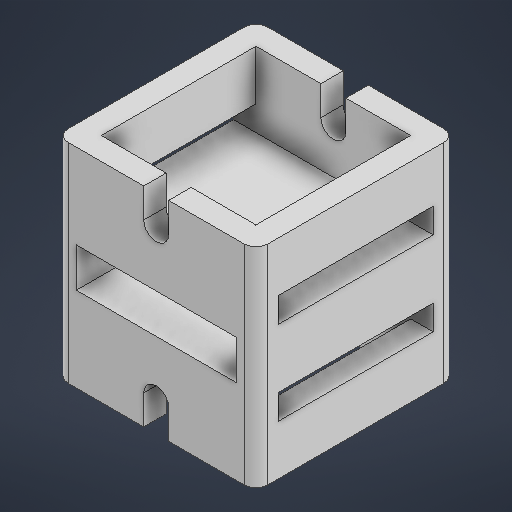
# Autodesk Inventor part: Part1
Saved by Autodesk Inventor 2026.1 (Build 301233000, 233)
## iProperties
Created: 2025-08-28
Part Number: Part1
Material: Generic
Document SubType Name: Modeling
Designer: usman
Density: 1 g/cm^3
Appearance: Default
Author: usman
Autodesk Inventor part; units mm, degrees
(part 1 of 2)
ref_plane "YZ Plane" through (0, 0, 0) normal (1, 0, 0) x (0, 1, 0)
ref_plane "XZ Plane" through (0, 0, 0) normal (0, 1, 0) x (-1, 0, 0)
ref_plane "XY Plane" through (0, 0, 0) normal (0, 0, 1) x (1, 0, 0)
sketch "Sketch1" plane through (0, 0, 0) normal (1, 0, 0) x (0, 1, 0)
  line L0 (-26.543, 25.4) -> (26.543, 25.4)
  line L1 (26.543, 25.4) -> (26.543, -25.4)
  line L2 (26.543, -25.4) -> (-26.543, -25.4)
  line L3 (-26.543, -25.4) -> (-26.543, 25.4)
  line L4 (-26.543, 25.4) -> (26.543, -25.4) construction
  line L5 (26.543, 25.4) -> (-26.543, -25.4) construction
  point P0 (0, 0)
  dimension "d0" = 53.086
  dimension "d1" = 50.8
  constraints: 12 end point, 2 midpoint, 2 parallel, 1 horizontal, 1 perpendicular
  measures "d0" distance of L1.end L2.end
  measures "d1" distance of L0.end L1.end
extrude "Extrusion1" add sketch "Sketch1" along normal blind 50.8
sketch "Sketch3" plane through (0, -26.543, -25.4) normal (0, -1, 0) x (1, 0, 0)
  line L0 (45.085, 5.715) -> (5.715, 5.715)
  line L1 (5.715, 5.715) -> (5.715, 45.085)
  line L2 (5.715, 45.085) -> (45.085, 45.085)
  line L3 (45.085, 45.085) -> (45.085, 5.715)
  line L4 (0, 0) -> (50.8, 0) projected
  line L5 (50.8, 50.8) -> (50.8, 0) projected
  point P0 (0, 25.4)
  dimension "d7" = 39.37
  dimension "d8" = 39.37
  dimension "d9" = 5.715
  dimension "d10" = 5.715
  constraints: 8 end point, 2 parallel, 1 horizontal, 1 perpendicular
  measures "d7" distance of L2.end L0.start
  measures "d8" distance of L0.start L0.end
  measures "d9" distance between parallel lines of L0 L4
  measures "d10" distance between parallel lines of L5 L3
extrude "Extrusion2" cut sketch "Sketch3" against normal blind 19.037
mirror "Mirror1" about plane through (0, 0, 0) normal (0, 1, 0) of "Extrusion2"
sketch "Sketch5" plane through (0, -26.543, 25.4) normal (0, 0, 1) x (1, 0, 0)
  line L0 (5.08, 31.543) -> (45.72, 31.543)
  line L1 (45.72, 31.543) -> (45.72, 21.543)
  line L2 (45.72, 21.543) -> (5.08, 21.543)
  line L3 (5.08, 21.543) -> (5.08, 31.543)
  line L4 (50.8, 53.086) -> (50.8, 0) projected
  line L5 (0, 53.086) -> (50.8, 53.086) projected
  point P0 (0, 26.543)
  dimension "d14" = 40.64
  dimension "d15" = 10
  dimension "d16" = 5.08
  dimension "d17" = 21.543
  constraints: 8 end point, 2 parallel, 1 horizontal, 1 perpendicular
  measures "d14" distance of L0.start L0.end
  measures "d15" distance of L2.end L0.start
  measures "d16" distance between parallel lines of L4 L1
  measures "d17" distance between parallel lines of L5 L0
extrude "Extrusion3" cut sketch "Sketch5" against normal through all
sketch "Sketch6" plane through (50.8, 0, 0) normal (1, 0, 0) x (0, 0, -1)
  line L0 (-19.685, 13.856) -> (19.685, 13.856)
  line L1 (19.685, 13.856) -> (19.685, 7.506)
  line L2 (19.685, 7.506) -> (-19.685, 7.506)
  line L3 (-19.685, 7.506) -> (-19.685, 13.856)
  line L4 (25.4, 26.543) -> (-25.4, 26.543) projected
  line L5 (-25.4, 26.543) -> (-25.4, -26.543) projected
  point P0 (0, 0)
  dimension "d20" = 39.37
  dimension "d21" = 6.35
  dimension "d22" = 12.687
  dimension "d23" = 5.715
  constraints: 8 end point, 2 parallel, 1 horizontal, 1 perpendicular
  measures "d20" distance of L0.start L0.end
  measures "d21" distance of L0.end L1.end
  measures "d22" distance between parallel lines of L4 L0
  measures "d23" distance between parallel lines of L5 L3
extrude "Extrusion4" cut sketch "Sketch6" against normal through all
mirror "Mirror2" about plane through (0, 0, 0) normal (0, 1, 0) of "Extrusion4"
sketch "Sketch7" plane through (0, -26.543, -25.4) normal (0, 0, -1) x (-1, 0, 0)
  line L0 (0, 53.086) -> (-50.8, 53.086) projected
  line L1 (-22.225, 53.086) -> (-22.225, 45.593)
  line L2 (-28.575, 53.086) -> (-28.575, 45.593)
  arc A0 (-28.575, 45.593) -> (-22.225, 45.593) centre (-25.4, 45.593) ccw
  point P0 (0, 26.543)
  point P1 (-25.4, 53.086)
  dimension "d26" = 7.493
  dimension "d27" = 7.493
  dimension "d28" = 3.175
  dimension "d29" = 3.175
  constraints: 4 end point, 2 point on circle, 2 point on line, 1 centre point, 1 midpoint, 1 perpendicular, 1 tangent, 1 vertical
  measures "d26" distance of L2.start L2.end
  measures "d27" distance of L1.start L1.end
  measures "d28" distance from line of L1 point (-25.4, 53.086)
  measures "d29" distance from line of point (-25.4, 53.086) L2
extrude "Extrusion5" cut sketch "Sketch7" against normal through all
mirror "Mirror3" about plane through (0, 0, 0) normal (0, 1, 0) of "Extrusion5"
fillet "Fillet2" radius 3 4 edges at (0, 0, -25.4) (0, 0, 25.4) (50.8, 0, -25.4) (50.8, 0, 25.4)
sketch "Sketch8" plane through (25.4, 19.05, -25.4) normal (0, 0, -1) x (-1, 0, 0)
  line L0 (-22.3221, -6.5134) -> (22.2832, -6.5134) construction
  line L1 (22.2832, -6.5134) -> (22.2832, -12.0545) construction
  line L2 (22.2832, -12.0545) -> (-22.3221, -12.0545) construction
  line L3 (-22.3221, -12.0545) -> (-22.3221, -6.5134) construction
  line L4 (-22.2875, -25.5953) -> (22.4563, -25.5953) construction
  line L5 (22.4563, -25.5953) -> (22.4563, -34.5995) construction
  line L6 (22.4563, -34.5995) -> (-22.2875, -34.5995) construction
  line L7 (-22.2875, -34.5995) -> (-22.2875, -25.5953) construction
  spline S0 degree 2 poles (-17.6545, -8.2254) (-17.325, -8.2955) (-17.1616, -8.4511) knots 0 0 0 1 1 1
  spline S1 degree 2 poles (-17.1616, -8.4511) (-16.9333, -8.6638) (-16.9333, -8.9751) knots 0 0 0 1 1 1
  spline S2 degree 2 poles (-16.9333, -8.9751) (-16.9333, -9.2111) (-17.2342, -9.6443) (-17.7556, -9.8441) (-18.2926, -9.8441) knots 0 0 0 1 2 3 3 3
  line L8 (-18.2926, -9.8441) -> (-19.7919, -9.8441)
  line L9 (-19.7919, -9.8441) -> (-19.7919, -9.7585)
  line L10 (-19.7919, -9.7585) -> (-19.6726, -9.7585)
  spline S3 degree 2 poles (-19.6726, -9.7585) (-19.4728, -9.7585) (-19.3872, -9.6314) knots 0 0 0 1 1 1
  spline S4 degree 2 poles (-19.3872, -9.6314) (-19.3328, -9.5483) (-19.3328, -9.2812) knots 0 0 0 1 1 1
  line L11 (-19.3328, -9.2812) -> (-19.3328, -7.2319)
  spline S5 degree 2 poles (-19.3328, -7.2319) (-19.3328, -6.9362) (-19.4002, -6.8584) knots 0 0 0 1 1 1
  spline S6 degree 2 poles (-19.4002, -6.8584) (-19.491, -6.7547) (-19.6726, -6.7547) knots 0 0 0 1 1 1
  line L12 (-19.6726, -6.7547) -> (-19.7919, -6.7547)
  line L13 (-19.7919, -6.7547) -> (-19.7919, -6.6691)
  line L14 (-19.7919, -6.6691) -> (-18.4197, -6.6691)
  spline S7 degree 2 poles (-18.4197, -6.6691) (-18.0358, -6.6691) (-17.8023, -6.7261) knots 0 0 0 1 1 1
  spline S8 degree 2 poles (-17.8023, -6.7261) (-17.4521, -6.8091) (-17.0812, -7.2397) (-17.0812, -7.5173) knots 0 0 0 1 2 2 2
  spline S9 degree 2 poles (-17.0812, -7.5173) (-17.0812, -7.7559) (-17.3717, -8.1346) (-17.6545, -8.2254) knots 0 0 0 1 2 2 2
  spline S10 degree 2 poles (-18.884, -9.6158) (-18.6116, -9.678) (-18.3445, -9.678) knots 0 0 0 1 1 1
  spline S11 degree 2 poles (-18.3445, -9.678) (-17.9191, -9.678) (-17.4703, -9.2967) (-17.4703, -9.0166) knots 0 0 0 1 2 2 2
  spline S12 degree 2 poles (-17.4703, -9.0166) (-17.4703, -8.8298) (-17.6778, -8.49) (-18.1344, -8.2929) (-18.469, -8.2929) knots 0 0 0 1 2 3 3 3
  spline S13 degree 2 poles (-18.469, -8.2929) (-18.6142, -8.2929) (-18.8217, -8.3033) (-18.884, -8.3136) knots 0 0 0 1 2 2 2
  line L15 (-18.884, -8.3136) -> (-18.884, -9.6158)
  spline S14 degree 2 poles (-18.884, -8.0983) (-18.7984, -8.1165) (-18.5753, -8.132) (-18.4404, -8.132) knots 0 0 0 1 2 2 2
  spline S15 degree 2 poles (-18.4404, -8.132) (-18.098, -8.132) (-17.753, -7.9842) (-17.5715, -7.6781) (-17.5715, -7.4991) knots 0 0 0 1 2 3 3 3
  spline S16 degree 2 poles (-17.5715, -7.4991) (-17.5715, -7.219) (-18.0254, -6.8247) (-18.4612, -6.8247) knots 0 0 0 1 2 2 2
  spline S17 degree 2 poles (-18.4612, -6.8247) (-18.6972, -6.8247) (-18.884, -6.8766) knots 0 0 0 1 1 1
  line L16 (-18.884, -6.8766) -> (-18.884, -8.0983)
  spline S18 degree 2 poles (-15.3095, -9.5328) (-15.639, -9.7896) (-15.7246, -9.8285) knots 0 0 0 1 1 1
  spline S19 degree 2 poles (-15.7246, -9.8285) (-15.8491, -9.8882) (-15.9917, -9.8882) knots 0 0 0 1 1 1
  spline S20 degree 2 poles (-15.9917, -9.8882) (-16.2148, -9.8882) (-16.5028, -9.5847) (-16.5028, -9.3356) knots 0 0 0 1 2 2 2
  spline S21 degree 2 poles (-16.5028, -9.3356) (-16.5028, -9.18) (-16.4327, -9.0633) knots 0 0 0 1 1 1
  spline S22 degree 2 poles (-16.4327, -9.0633) (-16.3367, -8.905) (-15.862, -8.6249) (-15.3095, -8.4226) knots 0 0 0 1 2 2 2
  line L17 (-15.3095, -8.4226) -> (-15.3095, -8.3396)
  spline S23 degree 2 poles (-15.3095, -8.3396) (-15.3095, -8.0179) (-15.5119, -7.7793) (-15.7064, -7.7793) knots 0 0 0 1 2 2 2
  spline S24 degree 2 poles (-15.7064, -7.7793) (-15.8517, -7.7793) (-15.9399, -7.8597) knots 0 0 0 1 1 1
  spline S25 degree 2 poles (-15.9399, -7.8597) (-16.0281, -7.9375) (-16.0281, -8.0413) knots 0 0 0 1 1 1
  line L18 (-16.0281, -8.0413) -> (-16.0229, -8.1761)
  spline S26 degree 2 poles (-16.0229, -8.1761) (-16.0229, -8.2851) (-16.1344, -8.4018) (-16.2226, -8.4018) knots 0 0 0 1 2 2 2
  spline S27 degree 2 poles (-16.2226, -8.4018) (-16.3082, -8.4018) (-16.4197, -8.2799) (-16.4197, -8.1736) knots 0 0 0 1 2 2 2
  spline S28 degree 2 poles (-16.4197, -8.1736) (-16.4197, -7.9738) (-16.0073, -7.6366) (-15.6364, -7.6366) knots 0 0 0 1 2 2 2
  spline S29 degree 2 poles (-15.6364, -7.6366) (-15.351, -7.6366) (-15.1695, -7.7326) knots 0 0 0 1 1 1
  spline S30 degree 2 poles (-15.1695, -7.7326) (-15.0294, -7.8052) (-14.9645, -7.9583) knots 0 0 0 1 1 1
  spline S31 degree 2 poles (-14.9645, -7.9583) (-14.923, -8.0594) (-14.923, -8.3707) knots 0 0 0 1 1 1
  line L19 (-14.923, -8.3707) -> (-14.923, -9.0996)
  spline S32 degree 2 poles (-14.923, -9.0996) (-14.923, -9.4057) (-14.8997, -9.5432) (-14.8452, -9.5899) (-14.8115, -9.5899) knots 0 0 0 1 2 3 3 3
  spline S33 degree 2 poles (-14.8115, -9.5899) (-14.7726, -9.5899) (-14.7441, -9.5743) knots 0 0 0 1 1 1
  spline S34 degree 2 poles (-14.7441, -9.5743) (-14.6948, -9.5432) (-14.5547, -9.4031) knots 0 0 0 1 1 1
  line L20 (-14.5547, -9.4031) -> (-14.5547, -9.5328)
  spline S35 degree 2 poles (-14.5547, -9.5328) (-14.8167, -9.8856) (-15.0553, -9.8856) knots 0 0 0 1 1 1
  spline S36 degree 2 poles (-15.0553, -9.8856) (-15.1721, -9.8856) (-15.3069, -9.7273) (-15.3095, -9.5328) knots 0 0 0 1 2 2 2
  line L21 (-15.3095, -9.3823) -> (-15.3095, -8.5652)
  spline S37 degree 2 poles (-15.3095, -8.5652) (-15.6623, -8.7053) (-15.7661, -8.765) knots 0 0 0 1 1 1
  spline S38 degree 2 poles (-15.7661, -8.765) (-15.9502, -8.8661) (-16.1085, -9.0918) (-16.1085, -9.2241) knots 0 0 0 1 2 2 2
  spline S39 degree 2 poles (-16.1085, -9.2241) (-16.1085, -9.3927) (-15.9087, -9.6158) (-15.7764, -9.6158) knots 0 0 0 1 2 2 2
  spline S40 degree 2 poles (-15.7764, -9.6158) (-15.6001, -9.6158) (-15.3095, -9.3823) knots 0 0 0 1 1 1
  line L22 (-13.0087, -7.6366) -> (-13.0087, -8.3681)
  line L23 (-13.0087, -8.3681) -> (-13.0865, -8.3681)
  spline S41 degree 2 poles (-13.0865, -8.3681) (-13.1747, -8.0231) (-13.4523, -7.7741) (-13.6676, -7.7741) knots 0 0 0 1 2 2 2
  spline S42 degree 2 poles (-13.6676, -7.7741) (-13.831, -7.7741) (-14.0333, -7.9479) (-14.0333, -8.0516) knots 0 0 0 1 2 2 2
  spline S43 degree 2 poles (-14.0333, -8.0516) (-14.0333, -8.1839) (-13.9581, -8.2773) knots 0 0 0 1 1 1
  spline S44 degree 2 poles (-13.9581, -8.2773) (-13.888, -8.3733) (-13.665, -8.4822) knots 0 0 0 1 1 1
  line L24 (-13.665, -8.4822) -> (-13.3226, -8.6482)
  spline S45 degree 2 poles (-13.3226, -8.6482) (-12.8479, -8.8791) (-12.8479, -9.2578) knots 0 0 0 1 1 1
  spline S46 degree 2 poles (-12.8479, -9.2578) (-12.8479, -9.5509) (-13.2888, -9.9089) (-13.5638, -9.9089) knots 0 0 0 1 2 2 2
  spline S47 degree 2 poles (-13.5638, -9.9089) (-13.7609, -9.9089) (-14.0126, -9.8389) knots 0 0 0 1 1 1
  spline S48 degree 2 poles (-14.0126, -9.8389) (-14.0904, -9.8155) (-14.1397, -9.8155) knots 0 0 0 1 1 1
  spline S49 degree 2 poles (-14.1397, -9.8155) (-14.1915, -9.8155) (-14.2227, -9.8752) knots 0 0 0 1 1 1
  line L25 (-14.2227, -9.8752) -> (-14.3005, -9.8752)
  line L26 (-14.3005, -9.8752) -> (-14.3005, -9.11)
  line L27 (-14.3005, -9.11) -> (-14.2227, -9.11)
  spline S50 degree 2 poles (-14.2227, -9.11) (-14.1578, -9.4394) (-13.7895, -9.7714) (-13.5586, -9.7714) knots 0 0 0 1 2 2 2
  spline S51 degree 2 poles (-13.5586, -9.7714) (-13.3978, -9.7714) (-13.1955, -9.5821) (-13.1955, -9.4472) knots 0 0 0 1 2 2 2
  spline S52 degree 2 poles (-13.1955, -9.4472) (-13.1955, -9.2864) (-13.4211, -9.0659) (-14.1008, -8.7313) (-14.2071, -8.5938) knots 0 0 0 1 2 3 3 3
  spline S53 degree 2 poles (-14.2071, -8.5938) (-14.3109, -8.4615) (-14.3109, -8.2566) knots 0 0 0 1 1 1
  spline S54 degree 2 poles (-14.3109, -8.2566) (-14.3109, -7.992) (-13.9477, -7.6366) (-13.6598, -7.6366) knots 0 0 0 1 2 2 2
  spline S55 degree 2 poles (-13.6598, -7.6366) (-13.5327, -7.6366) (-13.3537, -7.6911) knots 0 0 0 1 1 1
  spline S56 degree 2 poles (-13.3537, -7.6911) (-13.2344, -7.7248) (-13.1955, -7.7248) knots 0 0 0 1 1 1
  spline S57 degree 2 poles (-13.1955, -7.7248) (-13.1566, -7.7248) (-13.115, -7.6911) (-13.0865, -7.6366) knots 0 0 0 1 2 2 2
  line L28 (-13.0865, -7.6366) -> (-13.0087, -7.6366)
  spline S58 degree 2 poles (-12.1657, -8.5082) (-12.1683, -8.9855) (-11.9348, -9.2552) knots 0 0 0 1 1 1
  spline S59 degree 2 poles (-11.9348, -9.2552) (-11.6988, -9.5276) (-11.3823, -9.5276) knots 0 0 0 1 1 1
  spline S60 degree 2 poles (-11.3823, -9.5276) (-11.1722, -9.5276) (-10.8609, -9.2967) (-10.7546, -9.014) knots 0 0 0 1 2 2 2
  line L29 (-10.7546, -9.014) -> (-10.6819, -9.0607)
  spline S61 degree 2 poles (-10.6819, -9.0607) (-10.7312, -9.3823) (-11.2033, -9.9089) (-11.5613, -9.9089) knots 0 0 0 1 2 2 2
  spline S62 degree 2 poles (-11.5613, -9.9089) (-11.9478, -9.9089) (-12.4977, -9.3071) (-12.4977, -8.8013) knots 0 0 0 1 2 2 2
  spline S63 degree 2 poles (-12.4977, -8.8013) (-12.4977, -8.2514) (-11.9322, -7.6366) (-11.5068, -7.6366) knots 0 0 0 1 2 2 2
  spline S64 degree 2 poles (-11.5068, -7.6366) (-11.1462, -7.6366) (-10.6819, -8.1113) (-10.6819, -8.5082) knots 0 0 0 1 2 2 2
  line L30 (-10.6819, -8.5082) -> (-12.1657, -8.5082)
  line L31 (-12.1657, -8.3733) -> (-11.1696, -8.3733)
  spline S65 degree 2 poles (-11.1696, -8.3733) (-11.1826, -8.1684) (-11.2189, -8.0828) knots 0 0 0 1 1 1
  spline S66 degree 2 poles (-11.2189, -8.0828) (-11.2785, -7.9531) (-11.5094, -7.8026) (-11.6365, -7.8026) knots 0 0 0 1 2 2 2
  spline S67 degree 2 poles (-11.6365, -7.8026) (-11.831, -7.8026) (-12.1397, -8.1035) (-12.1657, -8.3733) knots 0 0 0 1 2 2 2
  line L32 (-7.385, -9.8441) -> (-8.6145, -7.1723)
  line L33 (-8.6145, -7.1723) -> (-8.6145, -9.2941)
  spline S68 degree 2 poles (-8.6145, -9.2941) (-8.6145, -9.5873) (-8.5523, -9.6599) knots 0 0 0 1 1 1
  spline S69 degree 2 poles (-8.5523, -9.6599) (-8.4641, -9.7585) (-8.2773, -9.7585) knots 0 0 0 1 1 1
  line L34 (-8.2773, -9.7585) -> (-8.1658, -9.7585)
  line L35 (-8.1658, -9.7585) -> (-8.1658, -9.8441)
  line L36 (-8.1658, -9.8441) -> (-9.2682, -9.8441)
  line L37 (-9.2682, -9.8441) -> (-9.2682, -9.7585)
  line L38 (-9.2682, -9.7585) -> (-9.1567, -9.7585)
  spline S70 degree 2 poles (-9.1567, -9.7585) (-8.9543, -9.7585) (-8.8713, -9.6365) knots 0 0 0 1 1 1
  spline S71 degree 2 poles (-8.8713, -9.6365) (-8.8195, -9.5613) (-8.8195, -9.2941) knots 0 0 0 1 1 1
  line L39 (-8.8195, -9.2941) -> (-8.8195, -7.219)
  spline S72 degree 2 poles (-8.8195, -7.219) (-8.8195, -7.0089) (-8.8662, -6.9129) knots 0 0 0 1 1 1
  spline S73 degree 2 poles (-8.8662, -6.9129) (-8.8999, -6.8454) (-9.0737, -6.7547) (-9.2682, -6.7547) knots 0 0 0 1 2 2 2
  line L40 (-9.2682, -6.7547) -> (-9.2682, -6.6691)
  line L41 (-9.2682, -6.6691) -> (-8.3681, -6.6691)
  line L42 (-8.3681, -6.6691) -> (-7.2164, -9.1541)
  line L43 (-7.2164, -9.1541) -> (-6.0802, -6.6691)
  line L44 (-6.0802, -6.6691) -> (-5.1853, -6.6691)
  line L45 (-5.1853, -6.6691) -> (-5.1853, -6.7547)
  line L46 (-5.1853, -6.7547) -> (-5.2943, -6.7547)
  spline S74 degree 2 poles (-5.2943, -6.7547) (-5.4992, -6.7547) (-5.5822, -6.8766) knots 0 0 0 1 1 1
  spline S75 degree 2 poles (-5.5822, -6.8766) (-5.6341, -6.9518) (-5.6341, -7.219) knots 0 0 0 1 1 1
  line L47 (-5.6341, -7.219) -> (-5.6341, -9.2941)
  spline S76 degree 2 poles (-5.6341, -9.2941) (-5.6341, -9.5873) (-5.5692, -9.6599) knots 0 0 0 1 1 1
  spline S77 degree 2 poles (-5.5692, -9.6599) (-5.481, -9.7585) (-5.2943, -9.7585) knots 0 0 0 1 1 1
  line L48 (-5.2943, -9.7585) -> (-5.1853, -9.7585)
  line L49 (-5.1853, -9.7585) -> (-5.1853, -9.8441)
  line L50 (-5.1853, -9.8441) -> (-6.5316, -9.8441)
  line L51 (-6.5316, -9.8441) -> (-6.5316, -9.7585)
  line L52 (-6.5316, -9.7585) -> (-6.4201, -9.7585)
  spline S78 degree 2 poles (-6.4201, -9.7585) (-6.2151, -9.7585) (-6.1347, -9.6365) knots 0 0 0 1 1 1
  spline S79 degree 2 poles (-6.1347, -9.6365) (-6.0828, -9.5613) (-6.0828, -9.2941) knots 0 0 0 1 1 1
  line L53 (-6.0828, -9.2941) -> (-6.0828, -7.1723)
  line L54 (-6.0828, -7.1723) -> (-7.3072, -9.8441)
  line L55 (-7.3072, -9.8441) -> (-7.385, -9.8441)
  spline S80 degree 2 poles (-3.7197, -9.5328) (-4.0492, -9.7896) (-4.1348, -9.8285) knots 0 0 0 1 1 1
  spline S81 degree 2 poles (-4.1348, -9.8285) (-4.2593, -9.8882) (-4.402, -9.8882) knots 0 0 0 1 1 1
  spline S82 degree 2 poles (-4.402, -9.8882) (-4.625, -9.8882) (-4.913, -9.5847) (-4.913, -9.3356) knots 0 0 0 1 2 2 2
  spline S83 degree 2 poles (-4.913, -9.3356) (-4.913, -9.18) (-4.8429, -9.0633) knots 0 0 0 1 1 1
  spline S84 degree 2 poles (-4.8429, -9.0633) (-4.747, -8.905) (-4.2723, -8.6249) (-3.7197, -8.4226) knots 0 0 0 1 2 2 2
  line L56 (-3.7197, -8.4226) -> (-3.7197, -8.3396)
  spline S85 degree 2 poles (-3.7197, -8.3396) (-3.7197, -8.0179) (-3.9221, -7.7793) (-4.1166, -7.7793) knots 0 0 0 1 2 2 2
  spline S86 degree 2 poles (-4.1166, -7.7793) (-4.2619, -7.7793) (-4.3501, -7.8597) knots 0 0 0 1 1 1
  spline S87 degree 2 poles (-4.3501, -7.8597) (-4.4383, -7.9375) (-4.4383, -8.0413) knots 0 0 0 1 1 1
  line L57 (-4.4383, -8.0413) -> (-4.4331, -8.1761)
  spline S88 degree 2 poles (-4.4331, -8.1761) (-4.4331, -8.2851) (-4.5446, -8.4018) (-4.6328, -8.4018) knots 0 0 0 1 2 2 2
  spline S89 degree 2 poles (-4.6328, -8.4018) (-4.7184, -8.4018) (-4.83, -8.2799) (-4.83, -8.1736) knots 0 0 0 1 2 2 2
  spline S90 degree 2 poles (-4.83, -8.1736) (-4.83, -7.9738) (-4.4175, -7.6366) (-4.0466, -7.6366) knots 0 0 0 1 2 2 2
  spline S91 degree 2 poles (-4.0466, -7.6366) (-3.7613, -7.6366) (-3.5797, -7.7326) knots 0 0 0 1 1 1
  spline S92 degree 2 poles (-3.5797, -7.7326) (-3.4396, -7.8052) (-3.3748, -7.9583) knots 0 0 0 1 1 1
  spline S93 degree 2 poles (-3.3748, -7.9583) (-3.3332, -8.0594) (-3.3332, -8.3707) knots 0 0 0 1 1 1
  line L58 (-3.3332, -8.3707) -> (-3.3332, -9.0996)
  spline S94 degree 2 poles (-3.3332, -9.0996) (-3.3332, -9.4057) (-3.3099, -9.5432) (-3.2554, -9.5899) (-3.2217, -9.5899) knots 0 0 0 1 2 3 3 3
  spline S95 degree 2 poles (-3.2217, -9.5899) (-3.1828, -9.5899) (-3.1543, -9.5743) knots 0 0 0 1 1 1
  spline S96 degree 2 poles (-3.1543, -9.5743) (-3.105, -9.5432) (-2.9649, -9.4031) knots 0 0 0 1 1 1
  line L59 (-2.9649, -9.4031) -> (-2.9649, -9.5328)
  spline S97 degree 2 poles (-2.9649, -9.5328) (-3.2269, -9.8856) (-3.4655, -9.8856) knots 0 0 0 1 1 1
  spline S98 degree 2 poles (-3.4655, -9.8856) (-3.5823, -9.8856) (-3.7172, -9.7273) (-3.7197, -9.5328) knots 0 0 0 1 2 2 2
  line L60 (-3.7197, -9.3823) -> (-3.7197, -8.5652)
  spline S99 degree 2 poles (-3.7197, -8.5652) (-4.0725, -8.7053) (-4.1763, -8.765) knots 0 0 0 1 1 1
  spline S100 degree 2 poles (-4.1763, -8.765) (-4.3605, -8.8661) (-4.5187, -9.0918) (-4.5187, -9.2241) knots 0 0 0 1 2 2 2
  spline S101 degree 2 poles (-4.5187, -9.2241) (-4.5187, -9.3927) (-4.319, -9.6158) (-4.1867, -9.6158) knots 0 0 0 1 2 2 2
  spline S102 degree 2 poles (-4.1867, -9.6158) (-4.0103, -9.6158) (-3.7197, -9.3823) knots 0 0 0 1 1 1
  spline S103 degree 2 poles (-2.2308, -9.0607) (-2.428, -8.9647) (-2.6381, -8.6223) (-2.6381, -8.4122) knots 0 0 0 1 2 2 2
  spline S104 degree 2 poles (-2.6381, -8.4122) (-2.6381, -8.0957) (-2.1582, -7.6366) (-1.7821, -7.6366) knots 0 0 0 1 2 2 2
  spline S105 degree 2 poles (-1.7821, -7.6366) (-1.476, -7.6366) (-1.2503, -7.7871) knots 0 0 0 1 1 1
  line L61 (-1.2503, -7.7871) -> (-0.7964, -7.7871)
  spline S106 degree 2 poles (-0.7964, -7.7871) (-0.6952, -7.7871) (-0.6615, -7.7974) (-0.6537, -7.813) knots 0 0 0 1 2 2 2
  spline S107 degree 2 poles (-0.6537, -7.813) (-0.6407, -7.8337) (-0.6407, -7.8882) knots 0 0 0 1 1 1
  spline S108 degree 2 poles (-0.6407, -7.8882) (-0.6407, -7.9479) (-0.6537, -7.9712) knots 0 0 0 1 1 1
  spline S109 degree 2 poles (-0.6537, -7.9712) (-0.6589, -7.9842) (-0.6952, -7.9972) (-0.7964, -7.9972) knots 0 0 0 1 2 2 2
  line L62 (-0.7964, -7.9972) -> (-1.0765, -7.9972)
  spline S110 degree 2 poles (-1.0765, -7.9972) (-0.9442, -8.1658) (-0.9442, -8.4278) knots 0 0 0 1 1 1
  spline S111 degree 2 poles (-0.9442, -8.4278) (-0.9442, -8.7287) (-1.4033, -9.1541) (-1.7898, -9.1541) knots 0 0 0 1 2 2 2
  spline S112 degree 2 poles (-1.7898, -9.1541) (-1.9481, -9.1541) (-2.1167, -9.1074) knots 0 0 0 1 1 1
  spline S113 degree 2 poles (-2.1167, -9.1074) (-2.2178, -9.1956) (-2.2905, -9.3279) (-2.2905, -9.3746) knots 0 0 0 1 2 2 2
  spline S114 degree 2 poles (-2.2905, -9.3746) (-2.2905, -9.4161) (-2.2127, -9.4913) (-2.1011, -9.5068) knots 0 0 0 1 2 2 2
  spline S115 degree 2 poles (-2.1011, -9.5068) (-2.0363, -9.5172) (-1.7717, -9.5224) knots 0 0 0 1 1 1
  spline S116 degree 2 poles (-1.7717, -9.5224) (-1.2892, -9.5354) (-1.1465, -9.5561) knots 0 0 0 1 1 1
  spline S117 degree 2 poles (-1.1465, -9.5561) (-0.9287, -9.5873) (-0.6693, -9.8492) (-0.6693, -10.0386) knots 0 0 0 1 2 2 2
  spline S118 degree 2 poles (-0.6693, -10.0386) (-0.6693, -10.3032) (-0.9183, -10.5341) knots 0 0 0 1 1 1
  spline S119 degree 2 poles (-0.9183, -10.5341) (-1.284, -10.8765) (-1.8729, -10.8765) knots 0 0 0 1 1 1
  spline S120 degree 2 poles (-1.8729, -10.8765) (-2.3242, -10.8765) (-2.6355, -10.6741) knots 0 0 0 1 1 1
  spline S121 degree 2 poles (-2.6355, -10.6741) (-2.8119, -10.5574) (-2.8119, -10.4303) knots 0 0 0 1 1 1
  spline S122 degree 2 poles (-2.8119, -10.4303) (-2.8119, -10.3732) (-2.7859, -10.3188) knots 0 0 0 1 1 1
  spline S123 degree 2 poles (-2.7859, -10.3188) (-2.747, -10.2306) (-2.6225, -10.0775) knots 0 0 0 1 1 1
  spline S124 degree 2 poles (-2.6225, -10.0775) (-2.6043, -10.0568) (-2.3839, -9.8259) knots 0 0 0 1 1 1
  spline S125 degree 2 poles (-2.3839, -9.8259) (-2.5032, -9.7533) (-2.6043, -9.6365) (-2.6043, -9.5639) knots 0 0 0 1 2 2 2
  spline S126 degree 2 poles (-2.6043, -9.5639) (-2.6043, -9.4835) (-2.4721, -9.263) (-2.2308, -9.0607) knots 0 0 0 1 2 2 2
  spline S127 degree 2 poles (-2.2542, -9.8441) (-2.3657, -9.9634) (-2.4772, -10.1683) (-2.4772, -10.2539) knots 0 0 0 1 2 2 2
  spline S128 degree 2 poles (-2.4772, -10.2539) (-2.4772, -10.3654) (-2.3424, -10.4485) knots 0 0 0 1 1 1
  spline S129 degree 2 poles (-2.3424, -10.4485) (-2.1063, -10.5937) (-1.6627, -10.5937) knots 0 0 0 1 1 1
  spline S130 degree 2 poles (-1.6627, -10.5937) (-1.2425, -10.5937) (-0.8405, -10.298) (-0.8405, -10.132) knots 0 0 0 1 2 2 2
  spline S131 degree 2 poles (-0.8405, -10.132) (-0.8405, -10.0101) (-0.9598, -9.9582) knots 0 0 0 1 1 1
  spline S132 degree 2 poles (-0.9598, -9.9582) (-1.0817, -9.9089) (-1.4423, -9.8985) knots 0 0 0 1 1 1
  spline S133 degree 2 poles (-1.4423, -9.8985) (-1.9714, -9.8856) (-2.2542, -9.8441) knots 0 0 0 1 1 1
  spline S134 degree 2 poles (-1.8236, -7.7481) (-1.9974, -7.7481) (-2.2308, -8.0231) (-2.2308, -8.3084) knots 0 0 0 1 2 2 2
  spline S135 degree 2 poles (-2.2308, -8.3084) (-2.2308, -8.6794) (-2.0726, -8.8817) knots 0 0 0 1 1 1
  spline S136 degree 2 poles (-2.0726, -8.8817) (-1.9507, -9.0373) (-1.7613, -9.0373) knots 0 0 0 1 1 1
  spline S137 degree 2 poles (-1.7613, -9.0373) (-1.5849, -9.0373) (-1.3541, -8.7702) (-1.3541, -8.4848) knots 0 0 0 1 2 2 2
  spline S138 degree 2 poles (-1.3541, -8.4848) (-1.3541, -8.1139) (-1.5149, -7.9038) knots 0 0 0 1 1 1
  spline S139 degree 2 poles (-1.5149, -7.9038) (-1.6342, -7.7481) (-1.8236, -7.7481) knots 0 0 0 1 1 1
  spline S140 degree 2 poles (0.2231, -8.0905) (0.5992, -7.6366) (0.9416, -7.6366) knots 0 0 0 1 1 1
  spline S141 degree 2 poles (0.9416, -7.6366) (1.1154, -7.6366) (1.367, -7.813) (1.4422, -8.0127) knots 0 0 0 1 2 2 2
  spline S142 degree 2 poles (1.4422, -8.0127) (1.4941, -8.1528) (1.4941, -8.4433) knots 0 0 0 1 1 1
  line L63 (1.4941, -8.4433) -> (1.4941, -9.359)
  spline S143 degree 2 poles (1.4941, -9.359) (1.4941, -9.5613) (1.5278, -9.6339) knots 0 0 0 1 1 1
  spline S144 degree 2 poles (1.5278, -9.6339) (1.5538, -9.6936) (1.6679, -9.7585) (1.8209, -9.7585) knots 0 0 0 1 2 2 2
  line L64 (1.8209, -9.7585) -> (1.8209, -9.8441)
  line L65 (1.8209, -9.8441) -> (0.7574, -9.8441)
  line L66 (0.7574, -9.8441) -> (0.7574, -9.7585)
  line L67 (0.7574, -9.7585) -> (0.8015, -9.7585)
  spline S145 degree 2 poles (0.8015, -9.7585) (0.952, -9.7585) (1.0713, -9.6677) (1.0946, -9.5795) knots 0 0 0 1 2 2 2
  spline S146 degree 2 poles (1.0946, -9.5795) (1.105, -9.5432) (1.105, -9.359) knots 0 0 0 1 1 1
  line L68 (1.105, -9.359) -> (1.105, -8.4822)
  spline S147 degree 2 poles (1.105, -8.4822) (1.105, -8.1891) (0.9546, -7.9245) (0.7756, -7.9245) knots 0 0 0 1 2 2 2
  spline S148 degree 2 poles (0.7756, -7.9245) (0.498, -7.9245) (0.2231, -8.228) knots 0 0 0 1 1 1
  line L69 (0.2231, -8.228) -> (0.2231, -9.359)
  spline S149 degree 2 poles (0.2231, -9.359) (0.2231, -9.5769) (0.249, -9.6288) knots 0 0 0 1 1 1
  spline S150 degree 2 poles (0.249, -9.6288) (0.2827, -9.6962) (0.3969, -9.7585) (0.5732, -9.7585) knots 0 0 0 1 2 2 2
  line L70 (0.5732, -9.7585) -> (0.5732, -9.8441)
  line L71 (0.5732, -9.8441) -> (-0.4929, -9.8441)
  line L72 (-0.4929, -9.8441) -> (-0.4929, -9.7585)
  line L73 (-0.4929, -9.7585) -> (-0.4462, -9.7585)
  spline S151 degree 2 poles (-0.4462, -9.7585) (-0.2802, -9.7585) (-0.166, -9.5924) (-0.166, -9.359) knots 0 0 0 1 2 2 2
  line L74 (-0.166, -9.359) -> (-0.166, -8.5626)
  spline S152 degree 2 poles (-0.166, -8.5626) (-0.166, -8.1787) (-0.2023, -8.0101) (-0.275, -7.9479) (-0.3346, -7.9479) knots 0 0 0 1 2 3 3 3
  spline S153 degree 2 poles (-0.3346, -7.9479) (-0.3995, -7.9479) (-0.4903, -7.9842) knots 0 0 0 1 1 1
  line L75 (-0.4903, -7.9842) -> (-0.5266, -7.8986)
  line L76 (-0.5266, -7.8986) -> (0.1219, -7.6366)
  line L77 (0.1219, -7.6366) -> (0.2231, -7.6366)
  line L78 (0.2231, -7.6366) -> (0.2231, -8.0905)
  spline S154 degree 2 poles (2.3553, -8.5082) (2.3527, -8.9855) (2.5862, -9.2552) knots 0 0 0 1 1 1
  spline S155 degree 2 poles (2.5862, -9.2552) (2.8222, -9.5276) (3.1387, -9.5276) knots 0 0 0 1 1 1
  spline S156 degree 2 poles (3.1387, -9.5276) (3.3488, -9.5276) (3.6601, -9.2967) (3.7664, -9.014) knots 0 0 0 1 2 2 2
  line L79 (3.7664, -9.014) -> (3.839, -9.0607)
  spline S157 degree 2 poles (3.839, -9.0607) (3.7898, -9.3823) (3.3177, -9.9089) (2.9597, -9.9089) knots 0 0 0 1 2 2 2
  spline S158 degree 2 poles (2.9597, -9.9089) (2.5732, -9.9089) (2.0233, -9.3071) (2.0233, -8.8013) knots 0 0 0 1 2 2 2
  spline S159 degree 2 poles (2.0233, -8.8013) (2.0233, -8.2514) (2.5887, -7.6366) (3.0142, -7.6366) knots 0 0 0 1 2 2 2
  spline S160 degree 2 poles (3.0142, -7.6366) (3.3747, -7.6366) (3.839, -8.1113) (3.839, -8.5082) knots 0 0 0 1 2 2 2
  line L80 (3.839, -8.5082) -> (2.3553, -8.5082)
  line L81 (2.3553, -8.3733) -> (3.3514, -8.3733)
  spline S161 degree 2 poles (3.3514, -8.3733) (3.3384, -8.1684) (3.3021, -8.0828) knots 0 0 0 1 1 1
  spline S162 degree 2 poles (3.3021, -8.0828) (3.2424, -7.9531) (3.0116, -7.8026) (2.8845, -7.8026) knots 0 0 0 1 2 2 2
  spline S163 degree 2 poles (2.8845, -7.8026) (2.6899, -7.8026) (2.3812, -8.1035) (2.3553, -8.3733) knots 0 0 0 1 2 2 2
  line L82 (4.7495, -6.9933) -> (4.7495, -7.6989)
  line L83 (4.7495, -7.6989) -> (5.2501, -7.6989)
  line L84 (5.2501, -7.6989) -> (5.2501, -7.8623)
  line L85 (5.2501, -7.8623) -> (4.7495, -7.8623)
  line L86 (4.7495, -7.8623) -> (4.7495, -9.2552)
  spline S164 degree 2 poles (4.7495, -9.2552) (4.7495, -9.4627) (4.8688, -9.608) (4.9622, -9.608) knots 0 0 0 1 2 2 2
  spline S165 degree 2 poles (4.9622, -9.608) (5.04, -9.608) (5.1879, -9.512) (5.2268, -9.4187) knots 0 0 0 1 2 2 2
  line L87 (5.2268, -9.4187) -> (5.3176, -9.4187)
  spline S166 degree 2 poles (5.3176, -9.4187) (5.2346, -9.6495) (4.9337, -9.8804) (4.7755, -9.8804) knots 0 0 0 1 2 2 2
  spline S167 degree 2 poles (4.7755, -9.8804) (4.6665, -9.8804) (4.459, -9.7611) (4.3604, -9.538) (4.3604, -9.3071) knots 0 0 0 1 2 3 3 3
  line L88 (4.3604, -9.3071) -> (4.3604, -7.8623)
  line L89 (4.3604, -7.8623) -> (4.0206, -7.8623)
  line L90 (4.0206, -7.8623) -> (4.0206, -7.7845)
  spline S168 degree 2 poles (4.0206, -7.7845) (4.1503, -7.7326) (4.4201, -7.4887) (4.5264, -7.3201) knots 0 0 0 1 2 2 2
  spline S169 degree 2 poles (4.5264, -7.3201) (4.5809, -7.2294) (4.6769, -6.9933) knots 0 0 0 1 1 1
  line L91 (4.6769, -6.9933) -> (4.7495, -6.9933)
  line L92 (9.3927, -6.5964) -> (9.4653, -7.6755)
  line L93 (9.4653, -7.6755) -> (9.3927, -7.6755)
  spline S170 degree 2 poles (9.3927, -7.6755) (9.2474, -7.1904) (8.7105, -6.7624) (8.3344, -6.7624) knots 0 0 0 1 2 2 2
  spline S171 degree 2 poles (8.3344, -6.7624) (8.0205, -6.7624) (7.5121, -7.0841) (7.219, -7.7871) (7.219, -8.311) knots 0 0 0 1 2 3 3 3
  spline S172 degree 2 poles (7.219, -8.311) (7.219, -8.7416) (7.4939, -9.3746) (8.049, -9.7118) (8.4018, -9.7118) knots 0 0 0 1 2 3 3 3
  spline S173 degree 2 poles (8.4018, -9.7118) (8.7105, -9.7118) (9.1826, -9.4472) (9.4653, -9.0529) knots 0 0 0 1 2 2 2
  line L94 (9.4653, -9.0529) -> (9.538, -9.0996)
  spline S174 degree 2 poles (9.538, -9.0996) (9.2993, -9.5224) (8.6638, -9.9167) (8.2254, -9.9167) knots 0 0 0 1 2 2 2
  spline S175 degree 2 poles (8.2254, -9.9167) (7.4368, -9.9167) (7.0037, -9.3305) knots 0 0 0 1 1 1
  spline S176 degree 2 poles (7.0037, -9.3305) (6.682, -8.8947) (6.682, -8.3058) knots 0 0 0 1 1 1
  spline S177 degree 2 poles (6.682, -8.3058) (6.682, -7.8312) (7.1074, -7.0348) (7.8545, -6.5964) (8.2954, -6.5964) knots 0 0 0 1 2 3 3 3
  spline S178 degree 2 poles (8.2954, -6.5964) (8.6379, -6.5964) (8.9725, -6.765) knots 0 0 0 1 1 1
  spline S179 degree 2 poles (8.9725, -6.765) (9.071, -6.8169) (9.1125, -6.8169) knots 0 0 0 1 1 1
  spline S180 degree 2 poles (9.1125, -6.8169) (9.1774, -6.8169) (9.2241, -6.7728) knots 0 0 0 1 1 1
  spline S181 degree 2 poles (9.2241, -6.7728) (9.2837, -6.708) (9.3097, -6.5964) knots 0 0 0 1 1 1
  line L95 (9.3097, -6.5964) -> (9.3927, -6.5964)
  spline S182 degree 2 poles (11.0684, -9.5328) (10.739, -9.7896) (10.6534, -9.8285) knots 0 0 0 1 1 1
  spline S183 degree 2 poles (10.6534, -9.8285) (10.5288, -9.8882) (10.3862, -9.8882) knots 0 0 0 1 1 1
  spline S184 degree 2 poles (10.3862, -9.8882) (10.1631, -9.8882) (9.8752, -9.5847) (9.8752, -9.3356) knots 0 0 0 1 2 2 2
  spline S185 degree 2 poles (9.8752, -9.3356) (9.8752, -9.18) (9.9452, -9.0633) knots 0 0 0 1 1 1
  spline S186 degree 2 poles (9.9452, -9.0633) (10.0412, -8.905) (10.5159, -8.6249) (11.0684, -8.4226) knots 0 0 0 1 2 2 2
  line L96 (11.0684, -8.4226) -> (11.0684, -8.3396)
  spline S187 degree 2 poles (11.0684, -8.3396) (11.0684, -8.0179) (10.8661, -7.7793) (10.6715, -7.7793) knots 0 0 0 1 2 2 2
  spline S188 degree 2 poles (10.6715, -7.7793) (10.5262, -7.7793) (10.4381, -7.8597) knots 0 0 0 1 1 1
  spline S189 degree 2 poles (10.4381, -7.8597) (10.3499, -7.9375) (10.3499, -8.0413) knots 0 0 0 1 1 1
  line L97 (10.3499, -8.0413) -> (10.355, -8.1761)
  spline S190 degree 2 poles (10.355, -8.1761) (10.355, -8.2851) (10.2435, -8.4018) (10.1553, -8.4018) knots 0 0 0 1 2 2 2
  spline S191 degree 2 poles (10.1553, -8.4018) (10.0697, -8.4018) (9.9582, -8.2799) (9.9582, -8.1736) knots 0 0 0 1 2 2 2
  spline S192 degree 2 poles (9.9582, -8.1736) (9.9582, -7.9738) (10.3706, -7.6366) (10.7415, -7.6366) knots 0 0 0 1 2 2 2
  spline S193 degree 2 poles (10.7415, -7.6366) (11.0269, -7.6366) (11.2085, -7.7326) knots 0 0 0 1 1 1
  spline S194 degree 2 poles (11.2085, -7.7326) (11.3485, -7.8052) (11.4134, -7.9583) knots 0 0 0 1 1 1
  spline S195 degree 2 poles (11.4134, -7.9583) (11.4549, -8.0594) (11.4549, -8.3707) knots 0 0 0 1 1 1
  line L98 (11.4549, -8.3707) -> (11.4549, -9.0996)
  spline S196 degree 2 poles (11.4549, -9.0996) (11.4549, -9.4057) (11.4782, -9.5432) (11.5327, -9.5899) (11.5664, -9.5899) knots 0 0 0 1 2 3 3 3
  spline S197 degree 2 poles (11.5664, -9.5899) (11.6053, -9.5899) (11.6339, -9.5743) knots 0 0 0 1 1 1
  spline S198 degree 2 poles (11.6339, -9.5743) (11.6832, -9.5432) (11.8232, -9.4031) knots 0 0 0 1 1 1
  line L99 (11.8232, -9.4031) -> (11.8232, -9.5328)
  spline S199 degree 2 poles (11.8232, -9.5328) (11.5612, -9.8856) (11.3226, -9.8856) knots 0 0 0 1 1 1
  spline S200 degree 2 poles (11.3226, -9.8856) (11.2059, -9.8856) (11.071, -9.7273) (11.0684, -9.5328) knots 0 0 0 1 2 2 2
  line L100 (11.0684, -9.3823) -> (11.0684, -8.5652)
  spline S201 degree 2 poles (11.0684, -8.5652) (10.7156, -8.7053) (10.6118, -8.765) knots 0 0 0 1 1 1
  spline S202 degree 2 poles (10.6118, -8.765) (10.4277, -8.8661) (10.2694, -9.0918) (10.2694, -9.2241) knots 0 0 0 1 2 2 2
  spline S203 degree 2 poles (10.2694, -9.2241) (10.2694, -9.3927) (10.4692, -9.6158) (10.6015, -9.6158) knots 0 0 0 1 2 2 2
  spline S204 degree 2 poles (10.6015, -9.6158) (10.7779, -9.6158) (11.0684, -9.3823) knots 0 0 0 1 1 1
  line L101 (13.3692, -7.6366) -> (13.3692, -8.3681)
  line L102 (13.3692, -8.3681) -> (13.2914, -8.3681)
  spline S205 degree 2 poles (13.2914, -8.3681) (13.2032, -8.0231) (12.9257, -7.7741) (12.7104, -7.7741) knots 0 0 0 1 2 2 2
  spline S206 degree 2 poles (12.7104, -7.7741) (12.5469, -7.7741) (12.3446, -7.9479) (12.3446, -8.0516) knots 0 0 0 1 2 2 2
  spline S207 degree 2 poles (12.3446, -8.0516) (12.3446, -8.1839) (12.4198, -8.2773) knots 0 0 0 1 1 1
  spline S208 degree 2 poles (12.4198, -8.2773) (12.4899, -8.3733) (12.713, -8.4822) knots 0 0 0 1 1 1
  line L103 (12.713, -8.4822) -> (13.0554, -8.6482)
  spline S209 degree 2 poles (13.0554, -8.6482) (13.53, -8.8791) (13.53, -9.2578) knots 0 0 0 1 1 1
  spline S210 degree 2 poles (13.53, -9.2578) (13.53, -9.5509) (13.0891, -9.9089) (12.8141, -9.9089) knots 0 0 0 1 2 2 2
  spline S211 degree 2 poles (12.8141, -9.9089) (12.617, -9.9089) (12.3654, -9.8389) knots 0 0 0 1 1 1
  spline S212 degree 2 poles (12.3654, -9.8389) (12.2875, -9.8155) (12.2383, -9.8155) knots 0 0 0 1 1 1
  spline S213 degree 2 poles (12.2383, -9.8155) (12.1864, -9.8155) (12.1553, -9.8752) knots 0 0 0 1 1 1
  line L104 (12.1553, -9.8752) -> (12.0774, -9.8752)
  line L105 (12.0774, -9.8752) -> (12.0774, -9.11)
  line L106 (12.0774, -9.11) -> (12.1553, -9.11)
  spline S214 degree 2 poles (12.1553, -9.11) (12.2201, -9.4394) (12.5884, -9.7714) (12.8193, -9.7714) knots 0 0 0 1 2 2 2
  spline S215 degree 2 poles (12.8193, -9.7714) (12.9801, -9.7714) (13.1825, -9.5821) (13.1825, -9.4472) knots 0 0 0 1 2 2 2
  spline S216 degree 2 poles (13.1825, -9.4472) (13.1825, -9.2864) (12.9568, -9.0659) (12.2772, -8.7313) (12.1708, -8.5938) knots 0 0 0 1 2 3 3 3
  spline S217 degree 2 poles (12.1708, -8.5938) (12.0671, -8.4615) (12.0671, -8.2566) knots 0 0 0 1 1 1
  spline S218 degree 2 poles (12.0671, -8.2566) (12.0671, -7.992) (12.4302, -7.6366) (12.7181, -7.6366) knots 0 0 0 1 2 2 2
  spline S219 degree 2 poles (12.7181, -7.6366) (12.8452, -7.6366) (13.0242, -7.6911) knots 0 0 0 1 1 1
  spline S220 degree 2 poles (13.0242, -7.6911) (13.1435, -7.7248) (13.1825, -7.7248) knots 0 0 0 1 1 1
  spline S221 degree 2 poles (13.1825, -7.7248) (13.2214, -7.7248) (13.2629, -7.6911) (13.2914, -7.6366) knots 0 0 0 1 2 2 2
  line L107 (13.2914, -7.6366) -> (13.3692, -7.6366)
  line L108 (14.591, -7.6366) -> (14.591, -9.359)
  spline S222 degree 2 poles (14.591, -9.359) (14.591, -9.5587) (14.648, -9.6936) (14.7648, -9.7585) (14.9152, -9.7585) knots 0 0 0 1 2 3 3 3
  line L109 (14.9152, -9.7585) -> (14.9152, -9.8441)
  line L110 (14.9152, -9.8441) -> (13.875, -9.8441)
  line L111 (13.875, -9.8441) -> (13.875, -9.7585)
  spline S223 degree 2 poles (13.875, -9.7585) (14.0307, -9.7585) (14.1396, -9.6988) (14.2019, -9.5587) (14.2019, -9.359) knots 0 0 0 1 2 3 3 3
  line L112 (14.2019, -9.359) -> (14.2019, -8.5341)
  spline S224 degree 2 poles (14.2019, -8.5341) (14.2019, -8.1865) (14.1811, -8.0828) knots 0 0 0 1 1 1
  spline S225 degree 2 poles (14.1811, -8.0828) (14.1656, -8.0075) (14.0929, -7.9479) (14.0333, -7.9479) knots 0 0 0 1 2 2 2
  spline S226 degree 2 poles (14.0333, -7.9479) (13.9684, -7.9479) (13.875, -7.9842) knots 0 0 0 1 1 1
  line L113 (13.875, -7.9842) -> (13.8413, -7.8986)
  line L114 (13.8413, -7.8986) -> (14.4872, -7.6366)
  line L115 (14.4872, -7.6366) -> (14.591, -7.6366)
  spline S227 degree 2 poles (14.3964, -6.5134) (14.495, -6.5134) (14.6325, -6.6509) (14.6325, -6.7495) knots 0 0 0 1 2 2 2
  spline S228 degree 2 poles (14.6325, -6.7495) (14.6325, -6.848) (14.495, -6.9881) (14.3964, -6.9881) knots 0 0 0 1 2 2 2
  spline S229 degree 2 poles (14.3964, -6.9881) (14.2979, -6.9881) (14.1578, -6.848) (14.1578, -6.7495) knots 0 0 0 1 2 2 2
  spline S230 degree 2 poles (14.1578, -6.7495) (14.1578, -6.6509) (14.2953, -6.5134) (14.3964, -6.5134) knots 0 0 0 1 2 2 2
  spline S231 degree 2 poles (15.8127, -8.0905) (16.1889, -7.6366) (16.5313, -7.6366) knots 0 0 0 1 1 1
  spline S232 degree 2 poles (16.5313, -7.6366) (16.705, -7.6366) (16.9567, -7.813) (17.0319, -8.0127) knots 0 0 0 1 2 2 2
  spline S233 degree 2 poles (17.0319, -8.0127) (17.0838, -8.1528) (17.0838, -8.4433) knots 0 0 0 1 1 1
  line L116 (17.0838, -8.4433) -> (17.0838, -9.359)
  spline S234 degree 2 poles (17.0838, -9.359) (17.0838, -9.5613) (17.1175, -9.6339) knots 0 0 0 1 1 1
  spline S235 degree 2 poles (17.1175, -9.6339) (17.1434, -9.6936) (17.2576, -9.7585) (17.4106, -9.7585) knots 0 0 0 1 2 2 2
  line L117 (17.4106, -9.7585) -> (17.4106, -9.8441)
  line L118 (17.4106, -9.8441) -> (16.3471, -9.8441)
  line L119 (16.3471, -9.8441) -> (16.3471, -9.7585)
  line L120 (16.3471, -9.7585) -> (16.3912, -9.7585)
  spline S236 degree 2 poles (16.3912, -9.7585) (16.5416, -9.7585) (16.661, -9.6677) (16.6843, -9.5795) knots 0 0 0 1 2 2 2
  spline S237 degree 2 poles (16.6843, -9.5795) (16.6947, -9.5432) (16.6947, -9.359) knots 0 0 0 1 1 1
  line L121 (16.6947, -9.359) -> (16.6947, -8.4822)
  spline S238 degree 2 poles (16.6947, -8.4822) (16.6947, -8.1891) (16.5442, -7.9245) (16.3652, -7.9245) knots 0 0 0 1 2 2 2
  spline S239 degree 2 poles (16.3652, -7.9245) (16.0877, -7.9245) (15.8127, -8.228) knots 0 0 0 1 1 1
  line L122 (15.8127, -8.228) -> (15.8127, -9.359)
  spline S240 degree 2 poles (15.8127, -9.359) (15.8127, -9.5769) (15.8387, -9.6288) knots 0 0 0 1 1 1
  spline S241 degree 2 poles (15.8387, -9.6288) (15.8724, -9.6962) (15.9865, -9.7585) (16.1629, -9.7585) knots 0 0 0 1 2 2 2
  line L123 (16.1629, -9.7585) -> (16.1629, -9.8441)
  line L124 (16.1629, -9.8441) -> (15.0968, -9.8441)
  line L125 (15.0968, -9.8441) -> (15.0968, -9.7585)
  line L126 (15.0968, -9.7585) -> (15.1435, -9.7585)
  spline S242 degree 2 poles (15.1435, -9.7585) (15.3095, -9.7585) (15.4236, -9.5924) (15.4236, -9.359) knots 0 0 0 1 2 2 2
  line L127 (15.4236, -9.359) -> (15.4236, -8.5626)
  spline S243 degree 2 poles (15.4236, -8.5626) (15.4236, -8.1787) (15.3873, -8.0101) (15.3147, -7.9479) (15.255, -7.9479) knots 0 0 0 1 2 3 3 3
  spline S244 degree 2 poles (15.255, -7.9479) (15.1902, -7.9479) (15.0994, -7.9842) knots 0 0 0 1 1 1
  line L128 (15.0994, -7.9842) -> (15.0631, -7.8986)
  line L129 (15.0631, -7.8986) -> (15.7116, -7.6366)
  line L130 (15.7116, -7.6366) -> (15.8127, -7.6366)
  line L131 (15.8127, -7.6366) -> (15.8127, -8.0905)
  spline S245 degree 2 poles (18.1577, -9.0607) (17.9605, -8.9647) (17.7504, -8.6223) (17.7504, -8.4122) knots 0 0 0 1 2 2 2
  spline S246 degree 2 poles (17.7504, -8.4122) (17.7504, -8.0957) (18.2303, -7.6366) (18.6064, -7.6366) knots 0 0 0 1 2 2 2
  spline S247 degree 2 poles (18.6064, -7.6366) (18.9125, -7.6366) (19.1382, -7.7871) knots 0 0 0 1 1 1
  line L132 (19.1382, -7.7871) -> (19.5921, -7.7871)
  spline S248 degree 2 poles (19.5921, -7.7871) (19.6933, -7.7871) (19.727, -7.7974) (19.7348, -7.813) knots 0 0 0 1 2 2 2
  spline S249 degree 2 poles (19.7348, -7.813) (19.7478, -7.8337) (19.7478, -7.8882) knots 0 0 0 1 1 1
  spline S250 degree 2 poles (19.7478, -7.8882) (19.7478, -7.9479) (19.7348, -7.9712) knots 0 0 0 1 1 1
  spline S251 degree 2 poles (19.7348, -7.9712) (19.7296, -7.9842) (19.6933, -7.9972) (19.5921, -7.9972) knots 0 0 0 1 2 2 2
  line L133 (19.5921, -7.9972) -> (19.312, -7.9972)
  spline S252 degree 2 poles (19.312, -7.9972) (19.4443, -8.1658) (19.4443, -8.4278) knots 0 0 0 1 1 1
  spline S253 degree 2 poles (19.4443, -8.4278) (19.4443, -8.7287) (18.9851, -9.1541) (18.5986, -9.1541) knots 0 0 0 1 2 2 2
  spline S254 degree 2 poles (18.5986, -9.1541) (18.4404, -9.1541) (18.2718, -9.1074) knots 0 0 0 1 1 1
  spline S255 degree 2 poles (18.2718, -9.1074) (18.1706, -9.1956) (18.098, -9.3279) (18.098, -9.3746) knots 0 0 0 1 2 2 2
  spline S256 degree 2 poles (18.098, -9.3746) (18.098, -9.4161) (18.1758, -9.4913) (18.2874, -9.5068) knots 0 0 0 1 2 2 2
  spline S257 degree 2 poles (18.2874, -9.5068) (18.3522, -9.5172) (18.6168, -9.5224) knots 0 0 0 1 1 1
  spline S258 degree 2 poles (18.6168, -9.5224) (19.0993, -9.5354) (19.2419, -9.5561) knots 0 0 0 1 1 1
  spline S259 degree 2 poles (19.2419, -9.5561) (19.4598, -9.5873) (19.7192, -9.8492) (19.7192, -10.0386) knots 0 0 0 1 2 2 2
  spline S260 degree 2 poles (19.7192, -10.0386) (19.7192, -10.3032) (19.4702, -10.5341) knots 0 0 0 1 1 1
  spline S261 degree 2 poles (19.4702, -10.5341) (19.1045, -10.8765) (18.5156, -10.8765) knots 0 0 0 1 1 1
  spline S262 degree 2 poles (18.5156, -10.8765) (18.0643, -10.8765) (17.753, -10.6741) knots 0 0 0 1 1 1
  spline S263 degree 2 poles (17.753, -10.6741) (17.5766, -10.5574) (17.5766, -10.4303) knots 0 0 0 1 1 1
  spline S264 degree 2 poles (17.5766, -10.4303) (17.5766, -10.3732) (17.6026, -10.3188) knots 0 0 0 1 1 1
  spline S265 degree 2 poles (17.6026, -10.3188) (17.6415, -10.2306) (17.766, -10.0775) knots 0 0 0 1 1 1
  spline S266 degree 2 poles (17.766, -10.0775) (17.7841, -10.0568) (18.0046, -9.8259) knots 0 0 0 1 1 1
  spline S267 degree 2 poles (18.0046, -9.8259) (17.8853, -9.7533) (17.7841, -9.6365) (17.7841, -9.5639) knots 0 0 0 1 2 2 2
  spline S268 degree 2 poles (17.7841, -9.5639) (17.7841, -9.4835) (17.9164, -9.263) (18.1577, -9.0607) knots 0 0 0 1 2 2 2
  spline S269 degree 2 poles (18.1343, -9.8441) (18.0228, -9.9634) (17.9112, -10.1683) (17.9112, -10.2539) knots 0 0 0 1 2 2 2
  spline S270 degree 2 poles (17.9112, -10.2539) (17.9112, -10.3654) (18.0461, -10.4485) knots 0 0 0 1 1 1
  spline S271 degree 2 poles (18.0461, -10.4485) (18.2822, -10.5937) (18.7257, -10.5937) knots 0 0 0 1 1 1
  spline S272 degree 2 poles (18.7257, -10.5937) (19.146, -10.5937) (19.548, -10.298) (19.548, -10.132) knots 0 0 0 1 2 2 2
  spline S273 degree 2 poles (19.548, -10.132) (19.548, -10.0101) (19.4287, -9.9582) knots 0 0 0 1 1 1
  spline S274 degree 2 poles (19.4287, -9.9582) (19.3068, -9.9089) (18.9462, -9.8985) knots 0 0 0 1 1 1
  spline S275 degree 2 poles (18.9462, -9.8985) (18.4171, -9.8856) (18.1343, -9.8441) knots 0 0 0 1 1 1
  spline S276 degree 2 poles (18.5649, -7.7481) (18.3911, -7.7481) (18.1577, -8.0231) (18.1577, -8.3084) knots 0 0 0 1 2 2 2
  spline S277 degree 2 poles (18.1577, -8.3084) (18.1577, -8.6794) (18.3159, -8.8817) knots 0 0 0 1 1 1
  spline S278 degree 2 poles (18.3159, -8.8817) (18.4378, -9.0373) (18.6272, -9.0373) knots 0 0 0 1 1 1
  spline S279 degree 2 poles (18.6272, -9.0373) (18.8036, -9.0373) (19.0344, -8.7702) (19.0344, -8.4848) knots 0 0 0 1 2 2 2
  spline S280 degree 2 poles (19.0344, -8.4848) (19.0344, -8.1139) (18.8736, -7.9038) knots 0 0 0 1 1 1
  spline S281 degree 2 poles (18.8736, -7.9038) (18.7543, -7.7481) (18.5649, -7.7481) knots 0 0 0 1 1 1
  spline S282 degree 2 poles (-7.6948, -27.0756) (-7.3654, -27.1456) (-7.202, -27.3012) knots 0 0 0 1 1 1
  spline S283 degree 2 poles (-7.202, -27.3012) (-6.9737, -27.5139) (-6.9737, -27.8252) knots 0 0 0 1 1 1
  spline S284 degree 2 poles (-6.9737, -27.8252) (-6.9737, -28.0613) (-7.2746, -28.4945) (-7.796, -28.6942) (-8.333, -28.6942) knots 0 0 0 1 2 3 3 3
  line L134 (-8.333, -28.6942) -> (-9.8323, -28.6942)
  line L135 (-9.8323, -28.6942) -> (-9.8323, -28.6086)
  line L136 (-9.8323, -28.6086) -> (-9.7129, -28.6086)
  spline S285 degree 2 poles (-9.7129, -28.6086) (-9.5132, -28.6086) (-9.4276, -28.4815) knots 0 0 0 1 1 1
  spline S286 degree 2 poles (-9.4276, -28.4815) (-9.3731, -28.3985) (-9.3731, -28.1313) knots 0 0 0 1 1 1
  line L137 (-9.3731, -28.1313) -> (-9.3731, -26.0821)
  spline S287 degree 2 poles (-9.3731, -26.0821) (-9.3731, -25.7864) (-9.4406, -25.7085) knots 0 0 0 1 1 1
  spline S288 degree 2 poles (-9.4406, -25.7085) (-9.5314, -25.6048) (-9.7129, -25.6048) knots 0 0 0 1 1 1
  line L138 (-9.7129, -25.6048) -> (-9.8323, -25.6048)
  line L139 (-9.8323, -25.6048) -> (-9.8323, -25.5192)
  line L140 (-9.8323, -25.5192) -> (-8.4601, -25.5192)
  spline S289 degree 2 poles (-8.4601, -25.5192) (-8.0762, -25.5192) (-7.8427, -25.5763) knots 0 0 0 1 1 1
  spline S290 degree 2 poles (-7.8427, -25.5763) (-7.4925, -25.6593) (-7.1216, -26.0899) (-7.1216, -26.3674) knots 0 0 0 1 2 2 2
  spline S291 degree 2 poles (-7.1216, -26.3674) (-7.1216, -26.6061) (-7.4121, -26.9848) (-7.6948, -27.0756) knots 0 0 0 1 2 2 2
  spline S292 degree 2 poles (-8.9244, -28.4659) (-8.652, -28.5282) (-8.3848, -28.5282) knots 0 0 0 1 1 1
  spline S293 degree 2 poles (-8.3848, -28.5282) (-7.9594, -28.5282) (-7.5107, -28.1469) (-7.5107, -27.8667) knots 0 0 0 1 2 2 2
  spline S294 degree 2 poles (-7.5107, -27.8667) (-7.5107, -27.68) (-7.7182, -27.3401) (-8.1747, -27.143) (-8.5093, -27.143) knots 0 0 0 1 2 3 3 3
  spline S295 degree 2 poles (-8.5093, -27.143) (-8.6546, -27.143) (-8.8621, -27.1534) (-8.9244, -27.1638) knots 0 0 0 1 2 2 2
  line L141 (-8.9244, -27.1638) -> (-8.9244, -28.4659)
  spline S296 degree 2 poles (-8.9244, -26.9485) (-8.8388, -26.9666) (-8.6157, -26.9822) (-8.4808, -26.9822) knots 0 0 0 1 2 2 2
  spline S297 degree 2 poles (-8.4808, -26.9822) (-8.1384, -26.9822) (-7.7934, -26.8343) (-7.6118, -26.5282) (-7.6118, -26.3493) knots 0 0 0 1 2 3 3 3
  spline S298 degree 2 poles (-7.6118, -26.3493) (-7.6118, -26.0691) (-8.0658, -25.6748) (-8.5016, -25.6748) knots 0 0 0 1 2 2 2
  spline S299 degree 2 poles (-8.5016, -25.6748) (-8.7376, -25.6748) (-8.9244, -25.7267) knots 0 0 0 1 1 1
  line L142 (-8.9244, -25.7267) -> (-8.9244, -26.9485)
  spline S300 degree 2 poles (-6.5405, -27.1248) (-6.5405, -26.5827) (-6.2137, -25.7993) (-5.9413, -25.6074) knots 0 0 0 1 2 2 2
  spline S301 degree 2 poles (-5.9413, -25.6074) (-5.7312, -25.4543) (-5.5055, -25.4543) knots 0 0 0 1 1 1
  spline S302 degree 2 poles (-5.5055, -25.4543) (-5.1398, -25.4543) (-4.8493, -25.8253) knots 0 0 0 1 1 1
  spline S303 degree 2 poles (-4.8493, -25.8253) (-4.4861, -26.287) (-4.4861, -27.0756) knots 0 0 0 1 1 1
  spline S304 degree 2 poles (-4.4861, -27.0756) (-4.4861, -27.6281) (-4.8052, -28.4011) (-5.298, -28.7487) (-5.5289, -28.7487) knots 0 0 0 1 2 3 3 3
  spline S305 degree 2 poles (-5.5289, -28.7487) (-5.9828, -28.7487) (-6.2863, -28.2117) knots 0 0 0 1 1 1
  spline S306 degree 2 poles (-6.2863, -28.2117) (-6.5405, -27.7604) (-6.5405, -27.1248) knots 0 0 0 1 1 1
  spline S307 degree 2 poles (-6.0814, -27.1845) (-6.0814, -27.8382) (-5.9206, -28.2532) knots 0 0 0 1 1 1
  spline S308 degree 2 poles (-5.9206, -28.2532) (-5.7857, -28.6008) (-5.5211, -28.6008) knots 0 0 0 1 1 1
  spline S309 degree 2 poles (-5.5211, -28.6008) (-5.394, -28.6008) (-5.1242, -28.3751) (-5.0542, -28.108) knots 0 0 0 1 2 2 2
  spline S310 degree 2 poles (-5.0542, -28.108) (-4.9453, -27.7059) (-4.9453, -26.9744) knots 0 0 0 1 1 1
  spline S311 degree 2 poles (-4.9453, -26.9744) (-4.9453, -26.4297) (-5.0568, -26.0691) knots 0 0 0 1 1 1
  spline S312 degree 2 poles (-5.0568, -26.0691) (-5.1424, -25.7993) (-5.2747, -25.6878) knots 0 0 0 1 1 1
  spline S313 degree 2 poles (-5.2747, -25.6878) (-5.3707, -25.61) (-5.5081, -25.61) knots 0 0 0 1 1 1
  spline S314 degree 2 poles (-5.5081, -25.61) (-5.6664, -25.61) (-5.7909, -25.7526) knots 0 0 0 1 1 1
  spline S315 degree 2 poles (-5.7909, -25.7526) (-5.9595, -25.9472) (-6.0814, -26.7798) (-6.0814, -27.1845) knots 0 0 0 1 2 2 2
  line L143 (-2.232, -25.5192) -> (-2.4136, -25.9161)
  line L144 (-2.4136, -25.9161) -> (-3.3681, -25.9161)
  line L145 (-3.3681, -25.9161) -> (-3.5782, -26.3415)
  spline S316 degree 2 poles (-3.5782, -26.3415) (-2.9583, -26.4323) (-2.5951, -26.8032) knots 0 0 0 1 1 1
  spline S317 degree 2 poles (-2.5951, -26.8032) (-2.2839, -27.1223) (-2.2839, -27.5528) knots 0 0 0 1 1 1
  spline S318 degree 2 poles (-2.2839, -27.5528) (-2.2839, -27.8019) (-2.4888, -28.2299) (-2.7975, -28.5282) (-2.9868, -28.619) knots 0 0 0 1 2 3 3 3
  spline S319 degree 2 poles (-2.9868, -28.619) (-3.2566, -28.7487) (-3.5393, -28.7487) knots 0 0 0 1 1 1
  spline S320 degree 2 poles (-3.5393, -28.7487) (-3.8273, -28.7487) (-4.0867, -28.5541) (-4.0867, -28.4374) knots 0 0 0 1 2 2 2
  spline S321 degree 2 poles (-4.0867, -28.4374) (-4.0867, -28.3725) (-3.9803, -28.2714) (-3.8973, -28.2714) knots 0 0 0 1 2 2 2
  spline S322 degree 2 poles (-3.8973, -28.2714) (-3.8376, -28.2714) (-3.7443, -28.3103) (-3.6353, -28.3881) knots 0 0 0 1 2 2 2
  spline S323 degree 2 poles (-3.6353, -28.3881) (-3.4589, -28.5074) (-3.2773, -28.51) knots 0 0 0 1 1 1
  spline S324 degree 2 poles (-3.2773, -28.51) (-3.005, -28.51) (-2.5873, -28.095) (-2.5873, -27.7967) knots 0 0 0 1 2 2 2